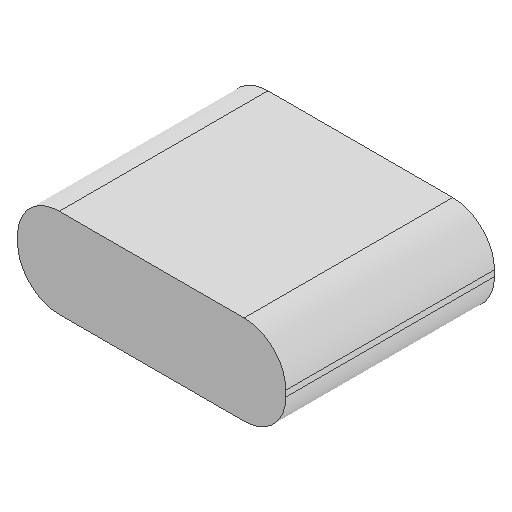
# Autodesk Inventor part: USB_C
Saved by Autodesk Inventor 2025.2 (Build 292293000, 293)
## iProperties
Created: 2025-03-09
Part Number: USB_C
Material: Generic
Document SubType Name: Modeling
Designer: ahorat
Density: 1 g/cm^3
Appearance: Default
Author: ahorat
Autodesk Inventor part; units mm, degrees
ref_plane "YZ Plane" through (0, 0, 0) normal (1, 0, 0) x (0, 1, 0)
ref_plane "XZ Plane" through (0, 0, 0) normal (0, 1, 0) x (-1, 0, 0)
ref_plane "XY Plane" through (0, 0, 0) normal (0, 0, 1) x (1, 0, 0)
sketch "Sketch1" plane through (0, 0, 0) normal (0, 0, 1) x (1, 0, 0)
  line L0 (-4.5, 0) -> (4.5, 0)
  line L1 (4.5, 0) -> (4.5, 3)
  line L2 (4.5, 3) -> (-4.5, 3)
  line L3 (-4.5, 3) -> (-4.5, 0)
  line L4 (-4.5, 0) -> (4.5, 3) construction
  line L5 (4.5, 0) -> (-4.5, 3) construction
  point P0 (0, 0)
  point P1 (0, 0)
  dimension "d0" = 9
  dimension "d1" = 3
  constraints: 12 end point, 2 parallel, 1 coincident, 1 horizontal, 1 midpoint, 1 perpendicular
  measures "d0" distance of L1.end L2.end
  measures "d1" distance of L0.end L1.end
extrude "Extrusion1" add sketch "Sketch1" along normal blind 7
fillet "Fillet1" radius 1.4 4 edges at (4.5, 3, 3.5) (-4.5, 3, 3.5) (-4.5, 0, 3.5) (4.5, 0, 3.5)
sketch "Sketch2" plane through (0, 0, 0) normal (0, 0, -1) x (-1, 0, 0)
  arc A0 (-4.5, 1.4) -> (-3.1, 0) centre (-3.1, 1.4) ccw projected
  line L0 (3.1, 0) -> (-3.1, 0) projected
  arc A1 (3.1, 0) -> (4.5, 1.4) centre (3.1, 1.4) ccw projected
  line L1 (4.5, 1.6) -> (4.5, 1.4) projected
  arc A2 (4.5, 1.6) -> (3.1, 3) centre (3.1, 1.6) ccw projected
  line L2 (-3.1, 3) -> (3.1, 3) projected
  arc A3 (-3.1, 3) -> (-4.5, 1.6) centre (-3.1, 1.6) ccw projected
  line L3 (-4.5, 1.4) -> (-4.5, 1.6) projected
  arc A4 (4.3, 1.6) -> (3.1, 2.8) centre (3.1, 1.6) ccw
  line L4 (4.3, 1.6) -> (4.3, 1.4)
  arc A5 (3.1, 0.2) -> (4.3, 1.4) centre (3.1, 1.4) ccw
  line L5 (3.1, 0.2) -> (-3.1, 0.2)
  arc A6 (-4.3, 1.4) -> (-3.1, 0.2) centre (-3.1, 1.4) ccw
  line L6 (-4.3, 1.4) -> (-4.3, 1.6)
  arc A7 (-3.1, 2.8) -> (-4.3, 1.6) centre (-3.1, 1.6) ccw
  line L7 (-3.1, 2.8) -> (3.1, 2.8)
  line L8 (-3.5, 1.85) -> (3.5, 1.85)
  line L9 (3.5, 1.85) -> (3.5, 1.15)
  line L10 (3.5, 1.15) -> (-3.5, 1.15)
  line L11 (-3.5, 1.15) -> (-3.5, 1.85)
  line L12 (-3.5, 1.85) -> (3.5, 1.15) construction
  line L13 (3.5, 1.85) -> (-3.5, 1.15) construction
  point P0 (0, 0)
  point P1 (0, 1.5)
  point P2 (4.5, 1.5)
  point P3 (0, 0)
  dimension "d5" = 0.2
  dimension "d6" = 7
  dimension "d7" = 0.7
  constraints: 20 end point, 8 point on circle, 4 centre point, 4 midpoint, 2 parallel, 1 horizontal, 1 horizontal alignment, 1 perpendicular, 1 vertical alignment, 7 other
  measures "d5" distance between parallel lines of L2 L7
  measures "d6" distance of L8.start L8.end
  measures "d7" distance between parallel lines of L10 L8
extrude "Extrusion2" cut sketch "Sketch2" against normal blind 6 contours L4 A5 L5 A6 L6 A7 L7 A4
fillet "Fillet2" radius 0.3 4 edges at (3.5, 1.15, 3) (3.5, 1.85, 3) (-3.5, 1.15, 3) (-3.5, 1.85, 3)
body "Solid1"
